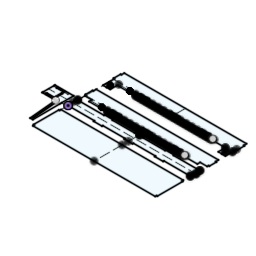
boitier_sysbee_CAD (Autodesk Fusion 360 design; units mm, degrees)
Autodesk Fusion 360 part; units mm, degrees
sketch "Esquisse1" plane through (0, 0, 0) normal (0, 1, 0) x (1, 0, 0)
  line L0 (0, 0) -> (0, 7)
  line L1 (0, 7) -> (-3, 7)
  line L2 (-3, 7) -> (-3, 17)
  line L3 (0, 0) -> (93.75, 0)
  line L4 (93.75, 0) -> (93.75, -3)
  line L5 (93.75, -3) -> (123.75, -3)
  line L6 (123.75, -3) -> (123.75, 0)
  line L7 (123.75, 0) -> (202.5, 0)
  line L8 (202.5, 0) -> (202.5, -3)
  line L9 (202.5, -3) -> (217.5, -3)
  line L10 (-3, 17) -> (438, 17) construction
  line L11 (217.5, -3) -> (217.5, 37) construction
  line L12 (202.5, 37) -> (217.5, 37)
  line L13 (-3, 27) -> (-3, 17)
  line L14 (202.5, 34) -> (202.5, 37)
  line L15 (123.75, 34) -> (202.5, 34)
  line L16 (0, 34) -> (0, 27)
  line L17 (0, 27) -> (-3, 27)
  line L18 (123.75, 37) -> (123.75, 34)
  line L19 (93.75, 37) -> (123.75, 37)
  line L20 (0, 34) -> (93.75, 34)
  line L21 (93.75, 34) -> (93.75, 37)
  line L22 (438, 7) -> (438, 17)
  line L23 (438, 27) -> (438, 17)
  line L24 (341.25, 37) -> (311.25, 37)
  line L25 (435, 34) -> (341.25, 34)
  line L26 (341.25, 0) -> (341.25, -3)
  line L27 (435, 27) -> (438, 27)
  line L28 (341.25, 34) -> (341.25, 37)
  line L29 (311.25, -3) -> (311.25, 0)
  line L30 (341.25, -3) -> (311.25, -3)
  line L31 (435, 34) -> (435, 27)
  line L32 (232.5, 34) -> (232.5, 37)
  line L33 (435, 0) -> (341.25, 0)
  line L34 (311.25, 0) -> (232.5, 0)
  line L35 (435, 7) -> (438, 7)
  line L36 (311.25, 37) -> (311.25, 34)
  line L37 (232.5, 0) -> (232.5, -3)
  line L38 (435, 0) -> (435, 7)
  line L39 (311.25, 34) -> (232.5, 34)
  line L40 (232.5, 37) -> (217.5, 37)
  line L41 (232.5, -3) -> (217.5, -3)
  point P0 (0, 34)
  point P1 (435, 34)
  point P2 (217.5, 37)
  point P3 (435, 0)
  dimension "d14" = 7
  dimension "plop" = 3
  dimension "d16" = 10
  dimension "d17" = 93.75
  dimension "d18" = 3
  dimension "d19" = 30
  dimension "d20" = 3
  dimension "d21" = 78.75
  dimension "d22" = 3
  dimension "d23" = 15
  dimension "d24" = 441
  dimension "d25" = 40
  constraint coincident L0.start L3.start
  constraint vertical L0
  constraint perpendicular L0 L1
  constraint perpendicular L1 L2
  constraint perpendicular L0 L3
  constraint perpendicular L3 L4
  constraint perpendicular L4 L5
  constraint perpendicular L5 L6
  constraint perpendicular L6 L7
  constraint perpendicular L7 L8
  constraint perpendicular L8 L9
  constraint perpendicular L2 L10
  constraint perpendicular L10 L11
  constraint symmetric L0.start L10 L16.start
  constraint symmetric L0.start L10 P0
  constraint symmetric L0.end L10 L16.end
  constraint symmetric L1.end L10 L13.start
  constraint symmetric L2.end L10 L13.end
  constraint symmetric L3.end L10 L20.end
  constraint symmetric L4.end L10 L19.start
  constraint symmetric L5.end L10 L18.start
  constraint symmetric L6.end L10 L15.start
  constraint symmetric L7.end L10 L14.start
  constraint symmetric L8.end L10 L12.start
  constraint symmetric L9.end L10 P2
  constraint symmetric L0.start L11 P3
  constraint symmetric L0.end L11 L35.start
  constraint symmetric L1.end L11 L22.start
  constraint symmetric L2.end L11 L10.end
  constraint symmetric L3.end L11 L26.start
  constraint symmetric L4.end L11 L26.end
  constraint symmetric L5.end L11 L29.start
  constraint symmetric L6.end L11 L29.end
  constraint symmetric L7.end L11 L34.end
  constraint symmetric L8.end L11 L37.end
  constraint symmetric L9.end L11 L41.end
  constraint symmetric P2 L11 L12.end
  constraint symmetric L11 L14.start L32.start
  constraint symmetric L11 L2.end L10.end
  constraint symmetric L11 P2 L12.end
  constraint symmetric L11 P0 P1
  constraint symmetric L11 L16.end L27.start
  constraint symmetric L11 L13.start L23.start
  constraint symmetric L11 L12.start L32.end
  constraint symmetric L11 L18.start L24.end
  constraint symmetric L11 L20.end L25.end
  constraint symmetric L11 L19.start L24.start
  constraint symmetric L11 L15.start L36.end
  measures "d14" distance of L0.start L0.end
  measures "plop" distance of L0.end L1.end
  measures "d16" distance of L1.end L2.end
  measures "d17" distance of L0.start L3.end
  measures "d18" distance of L3.end L4.end
  measures "d19" distance of L4.end L5.end
  measures "d20" distance of L5.end L6.end
  measures "d21" distance of L6.end L7.end
  measures "d22" distance of L7.end L8.end
  measures "d23" distance of L8.end L9.end
  measures "d24" distance of L2.end L10.end
  measures "d25" distance of L9.end P2
sketch "Esquisse2" plane through (0, 0, 0) normal (0, 1, 0) x (1, 0, 0)
  line L0 (0, 0) -> (0, 50) construction
  line L1 (0, 50) -> (0, 60) construction
  line L2 (0, 60) -> (25, 60)
  line L3 (25, 60) -> (25, 50)
  line L4 (410, 50) -> (410, 60)
  line L5 (410, 60) -> (435, 60)
  line L6 (435, 60) -> (435, 65)
  line L7 (435, 65) -> (438, 65)
  line L8 (438, 65) -> (438, 90)
  line L9 (438, 90) -> (435, 90)
  line L10 (435, 90) -> (435, 100)
  line L11 (435, 100) -> (0, 100)
  line L12 (0, 100) -> (0, 90)
  line L13 (0, 90) -> (-3, 90)
  line L14 (-3, 90) -> (-3, 65)
  line L15 (-3, 65) -> (0, 65)
  line L16 (0, 65) -> (0, 60)
  line L17 (-3, 65) -> (0, 65)
  line L18 (0, 60) -> (0, 62) construction
  line L19 (0, 62) -> (93.75, 62) construction
  line L20 (93.75, 62) -> (93.75, 65)
  line L21 (93.75, 65) -> (123.75, 65)
  line L22 (123.75, 65) -> (123.75, 62)
  line L23 (123.75, 62) -> (93.75, 62)
  line L24 (25, 50) -> (25, 55) construction
  line L25 (25, 55) -> (65, 55) construction
  line L26 (65, 55) -> (80, 55) construction
  line L27 (80, 55) -> (100, 55) construction
  line L28 (100, 55) -> (120, 55) construction
  line L29 (120, 55) -> (140, 55) construction
  line L30 (140, 55) -> (160, 55) construction
  line L31 (160, 55) -> (180, 55) construction
  line L32 (180, 55) -> (200, 55) construction
  line L33 (200, 55) -> (220, 55) construction
  line L34 (220, 55) -> (240, 55) construction
  line L35 (240, 55) -> (260, 55) construction
  line L36 (260, 55) -> (280, 55) construction
  line L37 (280, 55) -> (300, 55) construction
  line L38 (300, 55) -> (320, 55) construction
  line L39 (320, 55) -> (340, 55) construction
  line L40 (340, 55) -> (360, 55) construction
  line L41 (60, 55) -> (60, 50)
  line L42 (70, 55) -> (70, 50)
  arc A0 (70, 55) -> (60, 55) centre (65, 55) ccw
  arc A1 (90, 55) -> (80, 55) centre (85, 55) ccw
  line L43 (90, 55) -> (90, 50)
  line L44 (80, 55) -> (80, 50)
  arc A2 (110, 55) -> (100, 55) centre (105, 55) ccw
  line L45 (110, 55) -> (110, 50)
  line L46 (100, 55) -> (100, 50)
  arc A3 (130, 55) -> (120, 55) centre (125, 55) ccw
  line L47 (130, 55) -> (130, 50)
  line L48 (120, 55) -> (120, 50)
  arc A4 (150, 55) -> (140, 55) centre (145, 55) ccw
  line L49 (150, 55) -> (150, 50)
  line L50 (140, 55) -> (140, 50)
  arc A5 (170, 55) -> (160, 55) centre (165, 55) ccw
  line L51 (170, 55) -> (170, 50)
  line L52 (160, 55) -> (160, 50)
  arc A6 (190, 55) -> (180, 55) centre (185, 55) ccw
  line L53 (190, 55) -> (190, 50)
  line L54 (180, 55) -> (180, 50)
  arc A7 (210, 55) -> (200, 55) centre (205, 55) ccw
  line L55 (210, 55) -> (210, 50)
  line L56 (200, 55) -> (200, 50)
  arc A8 (230, 55) -> (220, 55) centre (225, 55) ccw
  line L57 (230, 55) -> (230, 50)
  line L58 (220, 55) -> (220, 50)
  arc A9 (250, 55) -> (240, 55) centre (245, 55) ccw
  line L59 (250, 55) -> (250, 50)
  line L60 (240, 55) -> (240, 50)
  arc A10 (270, 55) -> (260, 55) centre (265, 55) ccw
  line L61 (270, 55) -> (270, 50)
  line L62 (260, 55) -> (260, 50)
  arc A11 (290, 55) -> (280, 55) centre (285, 55) ccw
  line L63 (290, 55) -> (290, 50)
  line L64 (280, 55) -> (280, 50)
  arc A12 (310, 55) -> (300, 55) centre (305, 55) ccw
  line L65 (310, 55) -> (310, 50)
  line L66 (300, 55) -> (300, 50)
  arc A13 (330, 55) -> (320, 55) centre (325, 55) ccw
  line L67 (330, 55) -> (330, 50)
  line L68 (320, 55) -> (320, 50)
  arc A14 (350, 55) -> (340, 55) centre (345, 55) ccw
  line L69 (350, 55) -> (350, 50)
  line L70 (340, 55) -> (340, 50)
  arc A15 (370, 55) -> (360, 55) centre (365, 55) ccw
  line L71 (370, 55) -> (370, 50)
  line L72 (360, 55) -> (360, 50)
  line L73 (202.5, 65) -> (232.5, 65)
  line L74 (202.5, 62) -> (202.5, 65)
  line L75 (232.5, 62) -> (202.5, 62)
  line L76 (232.5, 65) -> (232.5, 62)
  line L77 (311.25, 65) -> (341.25, 65)
  line L78 (311.25, 62) -> (311.25, 65)
  line L79 (341.25, 62) -> (311.25, 62)
  line L80 (341.25, 65) -> (341.25, 62)
  line L81 (25, 50) -> (60, 50)
  line L82 (70, 50) -> (80, 50)
  line L83 (90, 50) -> (100, 50)
  line L84 (110, 50) -> (120, 50)
  line L85 (130, 50) -> (140, 50)
  line L86 (150, 50) -> (160, 50)
  line L87 (170, 50) -> (180, 50)
  line L88 (190, 50) -> (200, 50)
  line L89 (210, 50) -> (220, 50)
  line L90 (230, 50) -> (240, 50)
  line L91 (250, 50) -> (260, 50)
  line L92 (270, 50) -> (280, 50)
  line L93 (290, 50) -> (300, 50)
  line L94 (310, 50) -> (320, 50)
  line L95 (330, 50) -> (340, 50)
  line L96 (350, 50) -> (360, 50)
  line L97 (370, 50) -> (410, 50)
  dimension "d26" = 50
  dimension "d27" = 10
  dimension "d28" = 25
  dimension "d29" = 10
  dimension "d30" = 385
  dimension "d31" = 25
  dimension "d32" = 5
  dimension "d33" = 3
  dimension "d34" = 25
  dimension "d36" = 10
  dimension "d37" = 435
  dimension "d38" = 10
  dimension "d39" = 3
  dimension "d40" = 25
  dimension "d43" = 2
  dimension "d44" = 93.75
  dimension "d45" = 3
  dimension "d46" = 30
  dimension "d56" = 5
  dimension "d57" = 40
  dimension "d76" = 20
  dimension "d77" = 0
  dimension "d79" = 5
  dimension "d80" = 10
  dimension "d83" = 108.75
  dimension "d84" = 0
  dimension "d87" = 20
  dimension "d88" = 0
  dimension "d89" = 10
  constraint coincident L0.start origin
  constraint vertical L0
  constraint parallel L0 L1
  constraint perpendicular L0 L2
  constraint perpendicular L2 L3
  constraint perpendicular L4 L5
  constraint perpendicular L5 L6
  constraint perpendicular L6 L7
  constraint perpendicular L7 L8
  constraint perpendicular L8 L9
  constraint perpendicular L9 L10
  constraint perpendicular L8 L11
  constraint perpendicular L9 L12
  constraint perpendicular L12 L13
  constraint perpendicular L9 L14
  constraint perpendicular L12 L15
  constraint perpendicular L2 L16
  constraint perpendicular L2 L18
  constraint perpendicular L16 L19
  constraint perpendicular L19 L20
  constraint perpendicular L20 L21
  constraint perpendicular L21 L22
  constraint perpendicular L24 L25
  constraint coincident L25 L41.start
  constraint coincident L26 L42.start
  constraint coincident L25.end L26.start
  constraint perpendicular L41 L81
  constraint perpendicular L42 L82
  constraint horizontal L82
  constraint perpendicular L4 L97
  constraint horizontal L11
  constraint horizontal L26
  constraint horizontal L27
  constraint horizontal L28
  constraint horizontal L29
  constraint horizontal L30
  constraint horizontal L31
  constraint horizontal L32
  constraint horizontal L33
  constraint horizontal L34
  constraint horizontal L35
  constraint horizontal L36
  constraint horizontal L37
  constraint horizontal L38
  constraint horizontal L39
  constraint horizontal L40
  constraint horizontal L19.end L22.end
  constraint vertical L6.end L9.end
  constraint parallel L25 L81
  measures "d26" distance of L0.start L0.end
  measures "d27" distance of L0.end L1.end
  measures "d28" distance of L1.end L2.end
  measures "d29" distance of L2.end L3.end
  measures "d30" distance of L3.end L4.start
  measures "d31" distance of L4.end L5.end
  measures "d32" distance of L5.end L6.end
  measures "d33" distance of L6.end L7.end
  measures "d34" distance of L7.end L8.end
  measures "d36" distance of L9.end L10.end
  measures "d37" distance of L10.end L11.end
  measures "d38" distance of L11.end L12.end
  measures "d39" distance of L12.end L13.end
  measures "d40" distance of L13.end L14.end
  measures "d43" distance of L1.end L18.end
  measures "d44" distance of L18.end L19.end
  measures "d45" distance of L19.end L20.end
  measures "d46" distance of L20.end L21.end
  measures "d56" distance of L3.end L24.end
  measures "d57" distance of L24.end L25.end
  measures "d79" distance of L42.start L25.end
  measures "d80" distance of L41 L42
  measures "d89" distance of L4.start L4.end
sketch "face_laterale_boitier" plane through (0, 0, 0) normal (0, 1, 0) x (1, 0, 0)
  line L0 (0, 0) -> (0, -3) construction
  line L1 (0, -3) -> (-20, -3) construction
  line L2 (-20, -3) -> (-20, 37)
  line L3 (-86.5, 37) -> (-86.5, -3)
  line L4 (-47, -3) -> (-50, -3) construction
  line L5 (-50, -3) -> (-50, 37) construction
  line L6 (-50, 37) -> (-47, 37) construction
  line L7 (-47, 37) -> (-47, -3) construction
  line L8 (-50, 7) -> (-47, 7)
  line L9 (-47, 7) -> (-47, 27)
  line L10 (-47, 27) -> (-50, 27)
  line L11 (-50, 27) -> (-50, 7)
  line L12 (-48.5, 7) -> (-48.5, -3) construction
  line L13 (-50, 27) -> (-50, 34) construction
  line L14 (-50, 34) -> (-75, 34)
  line L15 (-75, 34) -> (-75, 37)
  line L16 (-75, 34) -> (-85, 34) construction
  line L17 (-85, 34) -> (-85, 37) construction
  line L18 (-75, 37) -> (-85, 37) construction
  line L19 (-50, 34) -> (-35, 34) construction
  line L20 (-20, 17) -> (-86.5, 17) construction
  line L21 (-85, 0) -> (-85, -3) construction
  line L22 (-75, -3) -> (-85, -3) construction
  line L23 (-75, 0) -> (-85, 0) construction
  line L24 (-50, 0) -> (-75, 0)
  line L25 (-75, 0) -> (-75, -3)
  line L26 (-50, 0) -> (-35, 0) construction
  line L27 (-50, 34) -> (-50, 37)
  line L28 (-50, 0) -> (-50, -3)
  line L29 (-20, 37) -> (-20, 40)
  line L30 (-20, 40) -> (-86.5, 40)
  line L31 (-86.5, 40) -> (-86.5, 37)
  line L32 (-20, -3) -> (-20, -9.6961)
  line L33 (-86.5, -6) -> (-86.5, -3)
  line L34 (-75, 37) -> (-50, 37)
  line L35 (-75, -3) -> (-50, -3)
  line L36 (-20, -9.6961) -> (-19.417, -105.9984)
  line L37 (-23.4041, -97.5414) -> (-26.391, -97.8209)
  line L38 (-26.391, -97.8209) -> (-34.7776, -8.2125)
  line L39 (-34.7776, -8.2125) -> (-31.7907, -7.933)
  line L40 (-31.7907, -7.933) -> (-23.4041, -97.5414)
  line L41 (-34.7776, -8.2125) -> (-35.2436, -3.2343) construction
  line L42 (-31.7907, -7.933) -> (-32.2566, -2.9547) construction
  line L43 (-26.391, -97.8209) -> (-25.9251, -102.7992) construction
  line L44 (-22.9381, -102.5196) -> (-25.9251, -102.7992) construction
  line L45 (-35.2436, -3.2343) -> (-32.2566, -2.9547) construction
  line L46 (-22.9381, -102.5196) -> (-23.4041, -97.5414) construction
  line L47 (-35, 34) -> (-35, 37) construction
  line L48 (-35, 37) -> (-50, 37) construction
  line L49 (-35, 0) -> (-35, -3) construction
  line L50 (-35, -3) -> (-50, -3) construction
  line L51 (-29.1355, -106.0572) -> (-38.5, -6)
  line L52 (-19.417, -105.9984) -> (-29.1355, -106.0572)
  line L53 (-86.5, -6) -> (-38.5, -6)
  line L54 (-50, -3) -> (-50, 0)
  line L55 (-50, 0) -> (-75, 0)
  line L56 (-75, -3) -> (-50, -3)
  line L57 (-75, 0) -> (-75, -3)
  dimension "d168" = 20
  dimension "d169" = 40
  dimension "d170" = 66.5
  dimension "d172" = 3
  dimension "d173" = 27
  dimension "d174" = 3
  dimension "d175" = 40
  dimension "d176" = 20
  dimension "d177" = 10
  dimension "d182" = 10
  dimension "d183" = 15
  dimension "d184" = 25
  dimension "d185" = 3
  dimension "d186" = 3
  dimension "d243" = 3
  dimension "d245" = 3
  dimension "d246" = 90
  dimension "d249" = 5
  dimension "d250" = 5
  dimension "d251" = 3.5
  dimension "d253" = 3
  dimension "d254" = 3
  dimension "d255" = 3
  dimension "d256" = 5
  dimension "d271" = 103
  dimension "d272" = 3.5
  dimension "d273" = 3.5
  dimension "d275" = 95.347
  dimension "d279" = 48
  constraint coincident L0.start origin
  constraint vertical L0
  constraint perpendicular L0 L1
  constraint perpendicular L1 L2
  constraint perpendicular L5 L6
  constraint perpendicular L4 L7
  constraint vertical L7
  constraint coincident L5 L8.start
  constraint perpendicular L5 L8
  constraint coincident L7 L9.end
  constraint coincident L5 L10.end
  constraint perpendicular L5 L10
  constraint vertical L11
  constraint vertical L9
  constraint midpoint L8 L12.start
  constraint midpoint L4 L12.end
  constraint perpendicular L10 L13
  constraint perpendicular L15 L16
  constraint perpendicular L5 L19
  constraint midpoint L2 L20.start
  constraint midpoint L3 L20.end
  constraint symmetric L5.end L20 L4.end
  constraint symmetric L13.end L20 L24.start
  constraint symmetric L15.end L20 L22.start
  constraint symmetric L14.end L20 L23.start
  constraint symmetric L16.end L20 L21.start
  constraint symmetric L17.end L20 L21.end
  constraint symmetric L19.end L20 L26.end
  constraint parallel L15 L27
  constraint perpendicular L14 L27
  constraint horizontal L5.end L15.end
  constraint perpendicular L29 L30
  constraint perpendicular L1 L32
  constraint vertical L33
  constraint parallel L38 L40
  constraint parallel L37 L39
  constraint perpendicular L39 L41
  constraint perpendicular L37 L43
  constraint parallel L37 L44
  constraint collinear L38 L41
  constraint perpendicular L41 L45
  constraint collinear L40 L42
  constraint perpendicular L37 L46
  constraint perpendicular L19 L47
  constraint parallel L20 L26
  constraint parallel L26 L50
  constraint parallel L28 L49
  constraint vertical L21.start L21.end
  constraint perpendicular L21 L22
  constraint perpendicular L3 L30
  constraint perpendicular L30 L31
  constraint parallel L38 L51
  constraint perpendicular L36 L52
  constraint coincident L51 L53.end
  constraint perpendicular L33 L53
  constraint parallel L30 L53
  measures "d168" distance of L0.end L1.end
  measures "d169" distance of L1.end L2.end
  measures "d170" distance of L2.end L3.start
  measures "d172" distance of L0.start L0.end
  measures "d173" distance of L1.end L4.start
  measures "d174" distance of L4.start L4.end
  measures "d175" distance of L4.end L5.end
  measures "d176" distance of L8.end L9.end
  measures "d177" distance of L12.start L12.end
  measures "d182" distance of L14.end L16.end
  measures "d183" distance of L13.end L19.end
  measures "d184" distance of L13.end L14.end
  measures "d185" distance of L5.end L13.end
  measures "d186" distance of L2.end L29.end
  measures "d243" distance of L3.end L33.start
  measures "d245" distance of L37.start L37.end
  measures "d246" distance of L37.start L39.end
  measures "d249" distance of L38.end L41.end
  measures "d250" distance of L37.end L43.end
  measures "d251" distance of L36 L44.start
  measures "d253" distance of L19.end L47.end
  measures "d254" distance of L26.end L49.end
  measures "d255" distance of L3.start L30.end
  measures "d256" angle of L36 L46
  measures "d271" distance of L1.end L36.end
  measures "d272" distance of L38 L51
  measures "d273" distance of L44.start L52
  measures "d275" angle of L51 L53
  measures "d279" distance of L33.start L51.end
extrude "Extrude1" add sketch "face_laterale_boitier" along normal blind 3 makes body 1
extrude "Extrude2" add sketch "Esquisse2" along normal blind 3 separate body makes body 2
extrude "Extrude3" add sketch "Esquisse1" along normal blind 3 separate body makes body 3
copy_body "Body->Comp1" bodies 1 removing the originals makes body 4 in component "face_gauche"
copy_body "Body->Comp1'" bodies 4 removing the originals makes body 5 in component "face_gauche (1)"
copy_body "Body->Comp2" bodies 2 removing the originals makes body 6 in component "face_arriere"
copy_body "Body->Comp3" bodies 3 removing the originals makes body 7 in component "support_carte"
extrude "Extrude1'" add sketch "Esquisse2" along normal blind 3 separate body makes body 8 in component "face_avant"
extrude "Extrude1''" add sketch "face_laterale_boitier" along normal blind 3 separate body makes body 9 in component "face_droite"
sketch "planche_envol" plane through (0, 0, 0) normal (0, 1, 0) x (1, 0, 0)
  line L0 (-3, -30) -> (0, -30)
  line L1 (0, -30) -> (0, -25)
  line L2 (0, -25) -> (217.5, -25)
  line L3 (-3, -30) -> (-3, -120)
  line L4 (-3, -120) -> (0, -120)
  line L5 (0, -120) -> (0, -125)
  line L6 (0, -125) -> (217.5, -125)
  line L7 (217.5, -25) -> (217.5, -125) construction
  line L8 (435, -25) -> (217.5, -25)
  line L9 (435, -30) -> (435, -25)
  line L10 (438, -30) -> (435, -30)
  line L11 (438, -30) -> (438, -120)
  line L12 (438, -120) -> (435, -120)
  line L13 (435, -120) -> (435, -125)
  line L14 (435, -125) -> (217.5, -125)
  line L15 (0, 0) -> (0, -25) construction
  dimension "d257" = 3
  dimension "d258" = 5
  dimension "d259" = 217.5
  dimension "d260" = 90
  dimension "d261" = 3
  dimension "d262" = 5
  dimension "d264" = 25
  constraint horizontal L0
  constraint perpendicular L0 L1
  constraint perpendicular L1 L2
  constraint perpendicular L0 L3
  constraint perpendicular L3 L4
  constraint perpendicular L0 L5
  constraint perpendicular L5 L6
  constraint symmetric L0.start L7 L10.start
  constraint symmetric L0.end L7 L9.start
  constraint symmetric L1.end L7 L8.start
  constraint symmetric L2.end L7 L8.end
  constraint symmetric L3.end L7 L11.end
  constraint symmetric L4.end L7 L12.end
  constraint symmetric L5.end L7 L13.end
  constraint symmetric L6.end L7 L14.end
  constraint equal L2 L6
  constraint coincident L15.start origin
  constraint vertical L15
  measures "d257" distance of L0.start L0.end
  measures "d258" distance of L0.end L1.end
  measures "d259" distance of L1.end L2.end
  measures "d260" distance of L0.start L3.end
  measures "d261" distance of L3.end L4.end
  measures "d262" distance of L4.end L5.end
  measures "d264" distance of L1.end L15.start
extrude "Extrude1'''" add sketch "planche_envol" along normal blind 3 separate body makes body 10 in component "planche_envol"
sketch "face_avant_boitier" plane through (0, 0, 0) normal (0, 1, 0) x (1, 0, 0)
  line L0 (0, 162) -> (93.75, 162) construction
  line L1 (100, 155) -> (120, 155) construction
  line L2 (340, 155) -> (340, 150)
  line L3 (123.75, 165) -> (123.75, 162)
  line L4 (320, 155) -> (320, 150)
  line L5 (80, 155) -> (100, 155) construction
  arc A0 (110, 155) -> (100, 155) centre (105, 155) ccw
  line L6 (90, 150) -> (100, 150)
  line L7 (90, 155) -> (90, 150)
  line L8 (202.5, 165) -> (232.5, 165)
  line L9 (190, 150) -> (200, 150)
  line L10 (25, 155) -> (65, 155) construction
  line L11 (300, 155) -> (300, 150)
  line L12 (130, 150) -> (140, 150)
  line L13 (310, 150) -> (320, 150)
  line L14 (300, 155) -> (320, 155) construction
  line L15 (290, 155) -> (290, 150)
  line L16 (60, 155) -> (60, 150)
  line L17 (190, 155) -> (190, 150)
  line L18 (160, 155) -> (160, 150)
  line L19 (80, 155) -> (80, 150)
  line L20 (25, 125) -> (25, 150)
  line L21 (200, 155) -> (220, 155) construction
  line L22 (120, 155) -> (120, 150)
  line L23 (232.5, 162) -> (202.5, 162)
  line L24 (330, 150) -> (340, 150)
  line L25 (65, 155) -> (80, 155) construction
  line L26 (341.25, 165) -> (341.25, 162)
  arc A1 (70, 155) -> (60, 155) centre (65, 155) ccw
  arc A2 (310, 155) -> (300, 155) centre (305, 155) ccw
  arc A3 (210, 155) -> (200, 155) centre (205, 155) ccw
  line L27 (150, 155) -> (150, 150)
  line L28 (120, 155) -> (140, 155) construction
  line L29 (330, 155) -> (330, 150)
  line L30 (370, 150) -> (410, 150)
  line L31 (0, 200) -> (0, 190)
  line L32 (0, 190) -> (-3, 190)
  line L33 (350, 155) -> (350, 150)
  line L34 (-3, 190) -> (-3, 165)
  line L35 (435, 165) -> (438, 165)
  line L36 (0, 125) -> (0, 162) construction
  line L37 (-3, 165) -> (0, 165)
  line L38 (0, 165) -> (0, 125)
  line L39 (438, 165) -> (438, 190)
  line L40 (93.75, 165) -> (123.75, 165)
  line L41 (435, 190) -> (435, 200)
  line L42 (438, 190) -> (435, 190)
  line L43 (310, 155) -> (310, 150)
  line L44 (0, 150) -> (0, 125) construction
  line L45 (311.25, 165) -> (341.25, 165)
  line L46 (350, 150) -> (360, 150)
  line L47 (320, 155) -> (340, 155) construction
  line L48 (-3, 165) -> (0, 165)
  arc A4 (230, 155) -> (220, 155) centre (225, 155) ccw
  line L49 (220, 155) -> (220, 150)
  line L50 (250, 150) -> (260, 150)
  line L51 (260, 155) -> (260, 150)
  line L52 (270, 150) -> (280, 150)
  line L53 (240, 155) -> (260, 155) construction
  line L54 (260, 155) -> (280, 155) construction
  arc A5 (290, 155) -> (280, 155) centre (285, 155) ccw
  line L55 (270, 155) -> (270, 150)
  line L56 (210, 150) -> (220, 150)
  line L57 (280, 155) -> (280, 150)
  line L58 (140, 155) -> (160, 155) construction
  line L59 (240, 155) -> (240, 150)
  line L60 (435, 200) -> (0, 200)
  line L61 (250, 155) -> (250, 150)
  line L62 (150, 150) -> (160, 150)
  arc A6 (150, 155) -> (140, 155) centre (145, 155) ccw
  line L63 (280, 155) -> (300, 155) construction
  line L64 (232.5, 165) -> (232.5, 162)
  line L65 (220, 155) -> (240, 155) construction
  line L66 (230, 150) -> (240, 150)
  arc A7 (270, 155) -> (260, 155) centre (265, 155) ccw
  line L67 (70, 150) -> (80, 150)
  line L68 (160, 155) -> (180, 155) construction
  line L69 (123.75, 162) -> (93.75, 162)
  arc A8 (170, 155) -> (160, 155) centre (165, 155) ccw
  line L70 (210, 155) -> (210, 150)
  arc A9 (250, 155) -> (240, 155) centre (245, 155) ccw
  line L71 (230, 155) -> (230, 150)
  arc A10 (130, 155) -> (120, 155) centre (125, 155) ccw
  arc A11 (90, 155) -> (80, 155) centre (85, 155) ccw
  line L72 (25, 150) -> (60, 150)
  line L73 (100, 155) -> (100, 150)
  line L74 (311.25, 162) -> (311.25, 165)
  line L75 (130, 155) -> (130, 150)
  line L76 (202.5, 162) -> (202.5, 165)
  line L77 (93.75, 162) -> (93.75, 165)
  line L78 (290, 150) -> (300, 150)
  line L79 (170, 155) -> (170, 150)
  line L80 (140, 155) -> (140, 150)
  line L81 (180, 155) -> (200, 155) construction
  line L82 (110, 150) -> (120, 150)
  line L83 (70, 155) -> (70, 150)
  arc A12 (190, 155) -> (180, 155) centre (185, 155) ccw
  line L84 (110, 155) -> (110, 150)
  line L85 (170, 150) -> (180, 150)
  arc A13 (330, 155) -> (320, 155) centre (325, 155) ccw
  line L86 (180, 155) -> (180, 150)
  line L87 (200, 155) -> (200, 150)
  line L88 (340, 155) -> (360, 155) construction
  line L89 (370, 155) -> (370, 150)
  line L90 (435, 150) -> (435, 165)
  line L91 (360, 155) -> (360, 150)
  arc A14 (350, 155) -> (340, 155) centre (345, 155) ccw
  arc A15 (370, 155) -> (360, 155) centre (365, 155) ccw
  line L92 (341.25, 162) -> (311.25, 162)
  line L93 (0, 125) -> (12.5, 125) construction
  line L94 (12.5, 137.5) -> (12.5, 125) construction
  line L95 (14, 137.5) -> (14, 125)
  line L96 (11, 137.5) -> (11, 125)
  arc A16 (14, 137.5) -> (11, 137.5) centre (12.5, 137.5) ccw
  line L97 (0, 125) -> (11, 125)
  line L98 (14, 125) -> (25, 125)
  line L99 (217.5, 200) -> (217.5, 150) construction
  line L100 (435, 165) -> (435, 125)
  line L101 (435, 125) -> (422.5, 125) construction
  line L102 (435, 125) -> (424, 125)
  line L103 (424, 137.5) -> (424, 125)
  line L104 (422.5, 137.5) -> (422.5, 125) construction
  line L105 (421, 137.5) -> (421, 125)
  arc A17 (424, 137.5) -> (421, 137.5) centre (422.5, 137.5) ccw
  line L106 (421, 125) -> (410, 125)
  line L107 (410, 125) -> (410, 150)
  line L108 (0, 150) -> (0, 0) construction
  point P0 (435, 150)
  dimension "d302" = 20
  dimension "d303" = 0
  dimension "d306" = 108.75
  dimension "d307" = 0
  dimension "d310" = 20
  dimension "d311" = 0
  dimension "d314" = 25
  dimension "d316" = 385
  dimension "d318" = 15
  dimension "d319" = 3
  dimension "d320" = 25
  dimension "d321" = 10
  dimension "d322" = 435
  dimension "d324" = 3
  dimension "d325" = 25
  dimension "d327" = 93.75
  dimension "d328" = 3
  dimension "d329" = 30
  dimension "d330" = 5
  dimension "d331" = 40
  dimension "d332" = 5
  dimension "d333" = 10
  dimension "d335" = 60
  dimension "d336" = 12
  dimension "d338" = 50
  dimension "d339" = 25
  dimension "d341" = 10
  dimension "d342" = 12.5
  dimension "d344" = 3
  dimension "d345" = 12.5
  dimension "d346" = 150
  constraint perpendicular L20 L97
  constraint perpendicular L35 L90
  constraint perpendicular L35 L39
  constraint perpendicular L39 L42
  constraint perpendicular L41 L42
  constraint perpendicular L39 L60
  constraint perpendicular L31 L42
  constraint perpendicular L31 L32
  constraint perpendicular L34 L42
  constraint perpendicular L31 L37
  constraint perpendicular L38 L97
  constraint perpendicular L36 L97
  constraint perpendicular L0 L38
  constraint perpendicular L0 L77
  constraint perpendicular L40 L77
  constraint perpendicular L3 L40
  constraint coincident L16.start L10
  constraint coincident A1.start L25
  constraint coincident L10.end L25.start
  constraint perpendicular L16 L72
  constraint perpendicular L67 L83
  constraint horizontal L67
  constraint horizontal L60
  constraint horizontal L25
  constraint horizontal L5
  constraint horizontal L1
  constraint horizontal L28
  constraint horizontal L58
  constraint horizontal L68
  constraint horizontal L81
  constraint horizontal L21
  constraint horizontal L65
  constraint horizontal L53
  constraint horizontal L54
  constraint horizontal L63
  constraint horizontal L14
  constraint horizontal L47
  constraint horizontal L88
  constraint horizontal L3.end L0.end
  constraint vertical L41.start L35.start
  constraint parallel L10 L72
  constraint vertical L44
  constraint horizontal L97
  constraint perpendicular L94 L97
  constraint coincident L94.start A16.centre
  constraint coincident L95.end L97
  constraint coincident L93 L96.end
  constraint tangent L95 A16
  constraint perpendicular L95 L97
  constraint tangent L96 A16
  constraint perpendicular L96 L97
  constraint collinear L97 L98
  constraint coincident L93.end L97
  constraint midpoint L60 L99.start
  constraint coincident L56 L99.end
  constraint perpendicular L56 L99
  constraint symmetric L36.start L99 L100.end
  constraint symmetric L20.end L99 L30.end
  constraint symmetric L20.start L99 L106.end
  constraint symmetric L37.end L99 L35.start
  constraint symmetric L93.end L99 L101.end
  constraint symmetric L94.start L99 L104.start
  constraint symmetric L95.start L99 L105.start
  constraint symmetric L95.end L99 L105.end
  constraint symmetric L96.start L99 L103.start
  constraint symmetric L96.end L99 L102.end
  constraint symmetric A16 L99 A17
  constraint coincident L108.end origin
  constraint parallel L44 L108
  constraint horizontal L44.start L20.end
  constraint symmetric L44.start L99 P0
  constraint horizontal L30
  constraint vertical L41.end L100.end
  measures "d314" distance of L36.start L20.start
  measures "d316" distance of L20.end L30.end
  measures "d318" distance of P0 L35.start
  measures "d319" distance of L35.end L35.start
  measures "d320" distance of L35.end L39.end
  measures "d321" distance of L41.end L41.start
  measures "d322" distance of L31.start L41.end
  measures "d324" distance of L32.end L31.end
  measures "d325" distance of L32.end L34.end
  measures "d327" distance of L0.start L0.end
  measures "d328" distance of L40.start L0.end
  measures "d329" distance of L40.start L3.start
  measures "d330" distance of L20.end L10.start
  measures "d331" distance of L10.end L10.start
  measures "d332" distance of A1.start L10.end
  measures "d333" distance of L16 L83
  measures "d335" distance of L16 L44
  measures "d336" distance of L44.start L0
  measures "d338" distance of L31.start L44.start
  measures "d339" distance of L20.end L20.start
  measures "d341" distance of L31.start L31.end
  measures "d342" distance of L93.end L94.start
  measures "d344" diameter of A16
  measures "d345" distance of L36.start L93.end
  measures "d346" distance of L44.start L108.end
component "face_gauche" placed x (1, 0, 0) y (0, 1, 0) z (0, 0, 1) at (0, 0, 0)
component "face_arriere" placed x (1, 0, 0) y (0, 0, 1) z (0, -1, 0) at (0, -62, -37)
component "support_carte" placed x (1, 0, 0) y (0, 1, 0) z (0, 0, 1) at (0, 0, 0)
component "face_avant" placed x (1, 0, 0) y (0, 0, 1) z (0, -1, 0) at (0, -62, 0)
component "face_droite" placed x (0, -1, 0) y (1, 0, 0) z (0, 0, 1) at (435, -47, 0)
component "planche_envol" placed x (1, 0, 0) y (0, 0.995649, 0.093185) z (0, -0.093185, 0.995649) at (0, -12.4138, -21.9365)
component "face_gauche (1)" placed x (0, -1, 0) y (1, 0, 0) z (0, 0, 1) at (-3, -47, 0) in component "face_gauche"
equation "plop = epaisseur"
equation "d18 = epaisseur"
equation "d20 = epaisseur"
equation "d22 = plop"
equation "d30 = 435 mm - 50 mm"
equation "d33 = epaisseur"
equation "d39 = epaisseur"
equation "d45 = epaisseur"
equation "epaisseur = 3 mm" comment "épaisseur du bois"
equation "d169 = 34 mm + 2 * epaisseur"
equation "d172 = epaisseur"
equation "d174 = epaisseur"
equation "d175 = 34 mm + 2 * epaisseur"
equation "d177 = 7 mm + epaisseur"
equation "d183 = 12 mm + epaisseur"
equation "d185 = epaisseur"
equation "d188 = epaisseur"
equation "d190 = epaisseur"
equation "d192 = epaisseur"
equation "d229 = epaisseur"
equation "d231 = epaisseur"
equation "d245 = epaisseur"
equation "d253 = epaisseur"
equation "d254 = epaisseur"
equation "d257 = epaisseur"
equation "d259 = ( 435 / 2 ) * 1 mm"
equation "d261 = epaisseur"
equation "d265 = epaisseur"
equation "d316 = 435 mm - 50 mm"
equation "d319 = epaisseur"
equation "d324 = epaisseur"
equation "d328 = epaisseur"
named bodies: "face_gauche", "face_arriere", "support_carte"
